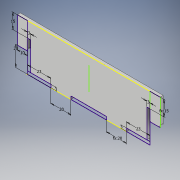
# Autodesk Inventor part: cham_back_v2
Saved by Autodesk Inventor 2017.2 (Build 212233000, 233)
## iProperties
Created: 2017-06-09
Part Number: cham_back_v2
Material: Generic
Document SubType Name: Modeling
Designer: SandeepSH
Density: 1 g/cm^3
Appearance: Default
Author: SandeepSH
Autodesk Inventor part; units mm, degrees
ref_plane "YZ Plane" through (0, 0, 0) normal (1, 0, 0) x (0, 1, 0)
ref_plane "XZ Plane" through (0, 0, 0) normal (0, 1, 0) x (-1, 0, 0)
ref_plane "XY Plane" through (0, 0, 0) normal (0, 0, 1) x (1, 0, 0)
sketch "Sketch1" plane through (0, 0, 0) normal (0, 0, 1) x (1, 0, 0)
  line L0 (0, 0) -> (121, 0)
  line L1 (121, 0) -> (121, 46)
  line L2 (121, 46) -> (0, 46)
  line L3 (0, 46) -> (0, 0)
  dimension "d0" = 121
  dimension "d1" = 46
  constraints: 8 end point, 2 parallel, 1 horizontal, 1 perpendicular
  measures "d0" distance of L2.end L1.end
  measures "d1" distance of L1.end L0.end
extrude "Extrusion1" add sketch "Sketch1" along normal blind 3
sketch "Sketch2" plane through (0, 0, 3) normal (0, 0, 1) x (1, 0, 0)
  line L0 (121, 0) -> (121, 46) projected
  line L1 (121, 0) -> (98, 0)
  line L2 (98, 0) -> (98, 3)
  line L3 (98, 3) -> (121, 3)
  line L4 (121, 3) -> (121, 0)
  line L5 (0, 0) -> (121, 0) projected
  line L6 (0, 0) -> (23, 0)
  line L7 (23, 0) -> (23, 3)
  line L8 (23, 3) -> (0, 3)
  line L9 (0, 3) -> (0, 0)
  line L10 (43, 0) -> (78, 0)
  line L11 (78, 0) -> (78, 3)
  line L12 (78, 3) -> (43, 3)
  line L13 (43, 3) -> (43, 0)
  line L14 (0, 3) -> (3, 3)
  line L15 (3, 3) -> (3, 31)
  line L16 (3, 31) -> (0, 31)
  line L17 (0, 31) -> (0, 3)
  line L18 (121, 46) -> (0, 46) projected
  line L19 (121, 3) -> (118, 3)
  line L20 (118, 3) -> (118, 31)
  line L21 (118, 31) -> (121, 31)
  line L22 (121, 31) -> (121, 3)
  dimension "d4" = 23
  dimension "d5" = 3
  dimension "d6" = 23
  dimension "d7" = 3
  dimension "d8" = 20
  dimension "d9" = 20
  dimension "d10" = 3
  dimension "d11" = 15
  dimension "d12" = 3
  dimension "d13" = 15
  constraints: 40 end point, 10 parallel, 5 horizontal, 5 perpendicular, 2 point on line
  measures "d4" distance of L2.end L3.end
  measures "d5" distance of L1.end L2.end
  measures "d6" distance of L8.end L7.end
  measures "d7" distance of L7.end L6.end
  measures "d8" distance between parallel lines of L13 L7
  measures "d9" distance between parallel lines of L2 L11
  measures "d10" distance of L16.end L15.end
  measures "d11" distance between parallel lines of L16 L18
  measures "d12" distance of L20.end L21.end
  measures "d13" distance between parallel lines of L21 L18
extrude "Extrusion2" cut sketch "Sketch2" against normal through all
sketch "Sketch3" plane through (0, 0, 3) normal (0, 0, 1) x (1, 0, 0)
  line L0 (121, 46) -> (0, 46) projected
  line L1 (0, 46) -> (-10, 46)
  line L2 (-10, 46) -> (-10, 20)
  line L3 (-10, 20) -> (0, 20)
  line L4 (0, 20) -> (0, 46)
  line L5 (23, 0) -> (43, 0) projected
  line L6 (60.5, 38.2025) -> (60.5, 15.3086)
  line L7 (121, 46) -> (131, 46)
  line L8 (131, 46) -> (131, 20)
  line L9 (131, 20) -> (121, 20)
  line L10 (121, 20) -> (121, 46)
  point P0 (0, 0)
  dimension "d16" = 10
  dimension "d17" = 20
  constraints: 18 end point, 3 symmetric about line, 2 parallel, 1 horizontal, 1 perpendicular, 1 vertical
  measures "d16" distance of L3.end L2.end
  measures "d17" distance between parallel lines of L5 L3
extrude "Extrusion3" add sketch "Sketch3" against normal blind 3
fillet "Fillet1" radius 2 4 edges at (0, 20, 1.5) (131, 20, 1.5) (121, 20, 1.5) (-10, 20, 1.5) curvature continuous yes
equation "\"d9\" = d8"
equation "\"d13\" = d11"
body "Solid1"
